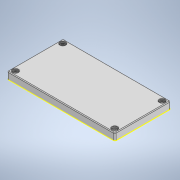
# Autodesk Inventor part: CustomLid_Rev3a
Saved by Autodesk Inventor 2021 (Build 250183000, 183)
## iProperties
Created: 2021-04-06
Part Number: CustomLid_Rev3a
Material: Generic
Document SubType Name: Modeling
Designer: James
Density: 1 g/cm^3
Appearance: Default
Author: James
Autodesk Inventor part; units mm, degrees
ref_plane "Ceiling" through (5.5793, 7, -57.7464) normal (0, -1, 0) x (1, 0, 0)
sketch "Sketch1" plane through (0, 0, 0) normal (0, 1, 0) x (-1, 0, 0)
  line L0 (103.9624, -60.4464) -> (103.9624, 16.5536) projected
  arc A0 (103.9624, 16.5536) -> (101.9624, 18.5536) centre (101.9624, 16.5536) ccw projected
  line L1 (101.9624, 18.5536) -> (-50.0376, 18.5536) projected
  arc A1 (-50.0376, 18.5536) -> (-52.0376, 16.5536) centre (-50.0376, 16.5536) ccw projected
  line L2 (-52.0376, 16.5536) -> (-52.0376, -60.4464) projected
  arc A2 (-52.0376, -60.4464) -> (-50.0376, -62.4464) centre (-50.0376, -60.4464) ccw projected
  line L3 (-50.0376, -62.4464) -> (101.9624, -62.4464) projected
  arc A3 (101.9624, -62.4464) -> (103.9624, -60.4464) centre (101.9624, -60.4464) ccw projected
  arc A4 (97.8999, -50.5293) -> (92.0453, -56.3839) centre (97.7805, -56.2644) ccw projected
  arc A5 (97.8833, -51.3291) -> (92.8451, -56.3672) centre (97.7805, -56.2644) ccw projected
  circle A6 centre (97.7805, -56.2644) radius 2.5 projected
  arc A7 (97.8999, -50.5293) -> (100.9624, -47.5299) centre (97.9624, -47.5299) ccw projected
  arc A8 (97.8833, -51.3291) -> (101.7624, -47.5299) centre (97.9624, -47.5299) ccw projected
  line L4 (100.9624, 3.6371) -> (100.9624, -47.5299) projected
  line L5 (101.7624, -47.5299) -> (101.7624, 3.6371) projected
  arc A9 (89.046, -60.2464) -> (92.8451, -56.3672) centre (89.046, -56.4464) ccw projected
  arc A10 (89.046, -59.4464) -> (92.0453, -56.3839) centre (89.046, -56.4464) ccw projected
  line L6 (89.046, -59.4464) -> (-37.1211, -59.4464) projected
  line L7 (-37.1211, -60.2464) -> (89.046, -60.2464) projected
  circle A11 centre (-45.8556, -56.2644) radius 2.5 projected
  arc A12 (-40.9203, -56.3672) -> (-45.9584, -51.3291) centre (-45.8556, -56.2644) ccw projected
  arc A13 (-40.1204, -56.3839) -> (-45.9751, -50.5293) centre (-45.8556, -56.2644) ccw projected
  arc A14 (-40.1204, -56.3839) -> (-37.1211, -59.4464) centre (-37.1211, -56.4464) ccw projected
  arc A15 (-40.9203, -56.3672) -> (-37.1211, -60.2464) centre (-37.1211, -56.4464) ccw projected
  arc A16 (-49.0376, -47.5299) -> (-45.9751, -50.5293) centre (-46.0376, -47.5299) ccw projected
  arc A17 (-49.8376, -47.5299) -> (-45.9584, -51.3291) centre (-46.0376, -47.5299) ccw projected
  line L8 (-49.0376, -47.5299) -> (-49.0376, 3.6371) projected
  line L9 (-49.8376, 3.6371) -> (-49.8376, -47.5299) projected
  circle A18 centre (-45.8556, 12.3716) radius 2.5 projected
  arc A19 (-45.9584, 7.4363) -> (-40.9203, 12.4745) centre (-45.8556, 12.3716) ccw projected
  arc A20 (-45.9751, 6.6365) -> (-40.1204, 12.4911) centre (-45.8556, 12.3716) ccw projected
  arc A21 (-45.9584, 7.4363) -> (-49.8376, 3.6371) centre (-46.0376, 3.6371) ccw projected
  arc A22 (-45.9751, 6.6365) -> (-49.0376, 3.6371) centre (-46.0376, 3.6371) ccw projected
  line L10 (-49.0376, -47.5299) -> (-49.0376, 3.6371) projected
  line L11 (-49.8376, 3.6371) -> (-49.8376, -47.5299) projected
  arc A23 (-37.1211, 16.3536) -> (-40.9203, 12.4745) centre (-37.1211, 12.5536) ccw projected
  arc A24 (-37.1211, 15.5536) -> (-40.1204, 12.4911) centre (-37.1211, 12.5536) ccw projected
  line L12 (89.046, 16.3536) -> (-37.1211, 16.3536) projected
  line L13 (-37.1211, 15.5536) -> (89.046, 15.5536) projected
  circle A25 centre (97.7805, 12.3716) radius 2.5 projected
  arc A26 (100.9624, 3.6371) -> (97.8999, 6.6365) centre (97.9624, 3.6371) ccw projected
  arc A27 (101.7624, 3.6371) -> (97.8833, 7.4363) centre (97.9624, 3.6371) ccw projected
  arc A28 (92.8451, 12.4745) -> (97.8833, 7.4363) centre (97.7805, 12.3716) ccw projected
  arc A29 (92.0453, 12.4911) -> (97.8999, 6.6365) centre (97.7805, 12.3716) ccw projected
  arc A30 (92.0453, 12.4911) -> (89.046, 15.5536) centre (89.046, 12.5536) ccw projected
  arc A31 (92.8451, 12.4745) -> (89.046, 16.3536) centre (89.046, 12.5536) ccw projected
  arc A32 (-48.3376, -47.5299) -> (-45.9897, -49.8294) centre (-46.0376, -47.5299) ccw
  arc A33 (-39.4206, -56.3985) -> (-45.9897, -49.8294) centre (-45.8556, -56.2644) ccw
  arc A34 (-39.4206, -56.3985) -> (-37.1211, -58.7464) centre (-37.1211, -56.4464) ccw
  line L14 (-37.1211, -58.7464) -> (89.046, -58.7464)
  arc A35 (89.046, -58.7464) -> (91.3455, -56.3985) centre (89.046, -56.4464) ccw
  arc A36 (97.9145, -49.8294) -> (91.3455, -56.3985) centre (97.7805, -56.2644) ccw
  arc A37 (97.9145, -49.8294) -> (100.2624, -47.5299) centre (97.9624, -47.5299) ccw
  line L15 (100.2624, -47.5299) -> (100.2624, 3.6371)
  arc A38 (100.2624, 3.6371) -> (97.9145, 5.9366) centre (97.9624, 3.6371) ccw
  arc A39 (91.3455, 12.5057) -> (97.9145, 5.9366) centre (97.7805, 12.3716) ccw
  arc A40 (91.3455, 12.5057) -> (89.046, 14.8536) centre (89.046, 12.5536) ccw
  line L16 (89.046, 14.8536) -> (-37.1211, 14.8536)
  arc A41 (-37.1211, 14.8536) -> (-39.4206, 12.5057) centre (-37.1211, 12.5536) ccw
  arc A42 (-45.9897, 5.9366) -> (-39.4206, 12.5057) centre (-45.8556, 12.3716) ccw
  arc A43 (-45.9897, 5.9366) -> (-48.3376, 3.6371) centre (-46.0376, 3.6371) ccw
  arc A44 (-45.9438, 8.1362) -> (-50.5376, 3.6371) centre (-46.0376, 3.6371) ccw
  arc A45 (-45.9438, 8.1362) -> (-41.6201, 12.4599) centre (-45.8556, 12.3716) ccw
  arc A46 (-37.1211, 17.0536) -> (-41.6201, 12.4599) centre (-37.1211, 12.5536) ccw
  line L17 (-37.1211, 17.0536) -> (89.046, 17.0536)
  arc A47 (93.545, 12.4599) -> (89.046, 17.0536) centre (89.046, 12.5536) ccw
  arc A48 (93.545, 12.4599) -> (97.8687, 8.1362) centre (97.7805, 12.3716) ccw
  arc A49 (102.4624, 3.6371) -> (97.8687, 8.1362) centre (97.9624, 3.6371) ccw
  line L18 (102.4624, 3.6371) -> (102.4624, -47.5299)
  arc A50 (97.8687, -52.0289) -> (102.4624, -47.5299) centre (97.9624, -47.5299) ccw
  arc A51 (97.8687, -52.0289) -> (93.545, -56.3527) centre (97.7805, -56.2644) ccw
  arc A52 (89.046, -60.9464) -> (93.545, -56.3527) centre (89.046, -56.4464) ccw
  line L19 (89.046, -60.9464) -> (-37.1211, -60.9464)
  arc A53 (-41.6201, -56.3527) -> (-37.1211, -60.9464) centre (-37.1211, -56.4464) ccw
  arc A54 (-41.6201, -56.3527) -> (-45.9438, -52.0289) centre (-45.8556, -56.2644) ccw
  arc A55 (-50.5376, -47.5299) -> (-45.9438, -52.0289) centre (-46.0376, -47.5299) ccw
  line L20 (-48.3376, -47.5299) -> (-48.3376, 3.6371)
  line L21 (-50.5376, 3.6371) -> (-50.5376, -47.5299)
  line L22 (-37.1211, 13.8536) -> (89.046, 13.8536)
  arc A56 (90.3457, 12.5265) -> (89.046, 13.8536) centre (89.046, 12.5536) ccw
  arc A57 (90.3457, 12.5265) -> (97.9354, 4.9368) centre (97.7805, 12.3716) ccw
  arc A58 (99.2624, 3.6371) -> (97.9354, 4.9368) centre (97.9624, 3.6371) ccw
  line L23 (99.2624, 3.6371) -> (99.2624, -47.5299)
  arc A59 (97.9354, -48.8296) -> (99.2624, -47.5299) centre (97.9624, -47.5299) ccw
  arc A60 (97.9354, -48.8296) -> (90.3457, -56.4193) centre (97.7805, -56.2644) ccw
  arc A61 (89.046, -57.7464) -> (90.3457, -56.4193) centre (89.046, -56.4464) ccw
  line L24 (89.046, -57.7464) -> (-37.1211, -57.7464)
  arc A62 (-38.4208, -56.4193) -> (-37.1211, -57.7464) centre (-37.1211, -56.4464) ccw
  arc A63 (-38.4208, -56.4193) -> (-46.0105, -48.8296) centre (-45.8556, -56.2644) ccw
  arc A64 (-47.3376, -47.5299) -> (-46.0105, -48.8296) centre (-46.0376, -47.5299) ccw
  line L25 (-47.3376, -47.5299) -> (-47.3376, 3.6371)
  arc A65 (-46.0105, 4.9368) -> (-47.3376, 3.6371) centre (-46.0376, 3.6371) ccw
  arc A66 (-46.0105, 4.9368) -> (-38.4208, 12.5265) centre (-45.8556, 12.3716) ccw
  arc A67 (-37.1211, 13.8536) -> (-38.4208, 12.5265) centre (-37.1211, 12.5536) ccw
  circle A68 centre (-32.1211, -53.4464) radius 1.25
  circle A69 centre (-43.0376, -21.9464) radius 1.25
  circle A70 centre (-32.1211, 9.5536) radius 1.25
  circle A71 centre (25.9624, 9.5536) radius 1.25
  circle A72 centre (25.9624, -53.4464) radius 1.25
  circle A73 centre (84.046, -53.4464) radius 1.25
  circle A74 centre (94.9624, -21.9464) radius 1.25
  circle A75 centre (84.046, 9.5536) radius 1.25
  circle A76 centre (-32.1211, 9.5536) radius 2.25
  circle A77 centre (25.9624, 9.5536) radius 2.25
  circle A78 centre (25.9624, -53.4464) radius 2.25
  circle A79 centre (-32.1211, -53.4464) radius 2.25
  circle A80 centre (-43.0376, -21.9464) radius 2.25
  circle A81 centre (84.046, 9.5536) radius 2.25
  circle A82 centre (94.9624, -21.9464) radius 2.25
  circle A83 centre (84.046, -53.4464) radius 2.25
  point P0 (0, 0)
  dimension "lid_gasket_delta" = 0.7
  dimension "d1" = 0.7
  dimension "d2" = 0.7
  dimension "d3" = 0.7
  dimension "d8" = 1
  constraints: 72 point on circle, 52 centre point, 24 end point, 2 parallel, 75 other
  measures "lid_gasket_delta" distance between parallel lines of L6 L14
  measures "d1" distance between parallel lines of L7 L19
  measures "d2" distance between parallel lines of L8 L20
  measures "d3" distance between parallel lines of L9 L21
  measures "d8" distance between parallel lines of L16 L22
extrude "Extrusion1" add sketch "Sketch1" along normal blind 10 contours A3 L3 A2 L2 A1 L1 A0 L0 | A4 A10 L6 A14 A13 A16 L8 A22 A20 A24 L13 A30 A29 A26 L4 A7 | A5 A9 L7 A15 A12 A17 L9 A21 A19 A23 L12 A31 A28 A27 L5 A8 | A6 | A11 | A18 | A25 | L20 A43 A42 A41 L16 A40 A39 A38 L15 A37 A36 A35 L14 A34 A33 A32 | A45 A46 L17 A47 A48 A49 L18 A50 A51 A52 L19 A53 A54 A55 L21 A44 | L22 A56 A57 A58 L23 A59 A60 A61 L24 A62 A63 A64 L25 A65 A66 A67 | A68 | A69 | A70 | A71 | A72 | A73 | A74 | A75 | A76 | A77 | A78 | A79 | A80 | A81 | A82 | A83
extrude "Extrusion2" cut sketch "Sketch1" along normal blind 7 from surface at 0 contours L22 A56 A57 A58 L23 A59 A60 A61 L24 A62 A63 A64 L25 A65 A66 A67 | A68 | A69 | A70 | A71 | A72 | A73 | A74 | A75 | A76 | A77 | A78 | A79 | A80 | A81 | A82 | A83
extrude "Extrusion3" cut sketch "Sketch1" along normal blind 2.5 contours A4 A10 L6 A14 A13 A16 L8 A22 A20 A24 L13 A30 A29 A26 L4 A7 | A5 A9 L7 A15 A12 A17 L9 A21 A19 A23 L12 A31 A28 A27 L5 A8 | A45 A46 L17 A47 A48 A49 L18 A50 A51 A52 L19 A53 A54 A55 L21 A44
ref_plane "Bottom Face" through (5.5793, 7, -57.7464) normal (0, -1, 0) x (1, 0, 0)
sketch "Sketch2" plane through (5.5793, 7, -57.7464) normal (0, -1, 0) x (1, 0, 0)
  circle A0 centre (26.5418, 67.3) radius 2.25 projected
  circle A1 centre (26.5418, 67.3) radius 1.25 projected
  circle A2 centre (37.4582, 35.8) radius 2.25 projected
  circle A3 centre (37.4582, 35.8) radius 1.25 projected
  circle A4 centre (26.5418, 4.3) radius 2.25 projected
  circle A5 centre (26.5418, 4.3) radius 1.25 projected
  circle A6 centre (-31.5418, 67.3) radius 2.25 projected
  circle A7 centre (-31.5418, 67.3) radius 1.25 projected
  circle A8 centre (-31.5418, 4.3) radius 2.25 projected
  circle A9 centre (-31.5418, 4.3) radius 1.25 projected
  circle A10 centre (-89.6253, 67.3) radius 2.25 projected
  circle A11 centre (-89.6253, 67.3) radius 1.25 projected
  circle A12 centre (-89.6253, 4.3) radius 2.25 projected
  circle A13 centre (-89.6253, 4.3) radius 1.25 projected
  circle A14 centre (-100.5418, 35.8) radius 2.25 projected
  circle A15 centre (-100.5418, 35.8) radius 1.25 projected
extrude "Extrusion4" add sketch "Sketch2" along normal blind 4 contours A0 | A1 | A2 | A3 | A4 | A5 | A6 | A7 | A8 | A9 | A10 | A11 | A12 | A13 | A14 | A15
extrude "Extrusion5" cut sketch "Sketch2" along normal blind 4 contours A1 | A3 | A5 | A7 | A9 | A11 | A13 | A15
fillet "Fillet1" radius 1.5 8 edges at (-86.296, 7, 9.5536) (-28.2124, 7, 9.5536) (29.8711, 7, 9.5536) (40.7876, 7, -21.9464) (29.8711, 7, -53.4464) (-28.2124, 7, -53.4464) (-86.296, 7, -53.4464) (-97.2124, 7, -21.9464)
ref_plane "Top Face" through (50.0376, 10, -62.4464) normal (0, 1, 0) x (-1, 0, 0)
sketch "Sketch3" plane through (50.0376, 10, -62.4464) normal (0, 1, 0) x (-1, 0, 0)
  circle A0 centre (147.818, 74.818) radius 2.5 projected
  circle A1 centre (4.182, 74.818) radius 2.5 projected
  circle A2 centre (4.182, 6.182) radius 2.5 projected
  circle A3 centre (147.818, 6.182) radius 2.5 projected
  point P0 (50.0376, 62.4464)
  point P1 (148.052, 74.8409)
  point P2 (148.052, 6.3093)
hole "Hole1" at (45.8556, 10, 12.3716) at (45.8556, 10, -56.2644) at (-98.0144, 10, 12.3945) at (-98.0144, 10, -56.1371) direction (0, -1, 0) diameter 4 end through all counterbore diameter 7.5 counterbore depth 2.5
fillet "Fillet2" radius 0.5 4 edges at (45.8556, 10, 8.6216) (45.8556, 10, -60.0144) (-98.0144, 10, 8.6445) (-98.0144, 10, -59.8871)
fillet "Fillet3" radius 0.5 4 edges at (45.8556, 7.5, 8.6216) (45.8556, 7.5, -60.0144) (-98.0144, 7.5, 8.6445) (-98.0144, 7.5, -59.8871) inverted yes
ref_plane "Inspection Plane" through (45.8556, 0, 12.3716) normal (0, 0, 1) x (1, 0, 0)
sketch "Sketch4" plane through (45.8556, 0, 12.3716) normal (0, 0, 1) x (1, 0, 0)
  point P0 (-45.8556, 0)
fillet "Fillet4" radius 1 8 edges at (51.4518, 10, 17.9678) (52.0376, 10, -21.9464) (51.4518, 10, -61.8606) (-25.9624, 10, -62.4464) (-103.3766, 10, -61.8606) (-103.9624, 10, -21.9464) (-103.3766, 10, 17.9678) (-25.9624, 10, 18.5536)
sketch "Sketch5" plane through (5.5793, 7, -57.7464) normal (0, -1, 0) x (1, 0, 0)
  line L0 (-84.1448, 70.2927) -> (6.5043, 70.2927) construction
  line L1 (6.5043, 70.2927) -> (6.5043, 55.3746) construction
  line L2 (6.5043, 55.3746) -> (-84.1448, 55.3746) construction
  line L3 (-84.1448, 55.3746) -> (-84.1448, 70.2927) construction
  point P0 (-5.5793, 57.7464)
  constraints: 2 other
equation "\"d1\" = lid_gasket_delta"
equation "\"d2\" = lid_gasket_delta"
equation "\"d3\" = lid_gasket_delta"
equation "\"d8\" = min_wall_width"
equation "\"d6\" = lid_height - wall_thickness"
equation "\"d12\" = pem_height"
equation "\"d14\" = pem_height"
equation "\"d16\" = PEM_fillet"
equation "\"d18\" = lid_screw_d"
equation "\"d23\" = pem_height"
equation "\"d30\" = bottom_fillet"
equation "\"wall_thickness\" = wall_thickness_1"
equation "\"min_wall_width\" = 1"
equation "\"lid_height\" = 10"
equation "\"pem_height\" = 4"
equation "\"PEM_fillet\" = 1.5"
equation "\"lid_screw_d\" = 4"
equation "\"bottom_fillet\" = 1"
equation "\"wall_thickness_1\" = 3"
body "Solid1"
